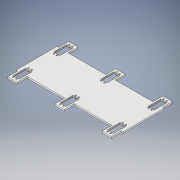
# Autodesk Inventor part: Body_Top
Saved by Autodesk Inventor 2017 (Build 210142000, 142)
## iProperties
Created: 2017-01-25
Part Number: Body_Top
Material: Generic
Document SubType Name: Modeling
Designer: Alexander Miller
Density: 1 g/cm^3
Appearance: Default
material_thickness: 5,000 mm
body_width: 130,000 mm
leg_distance: 120,000 mm
Author: Alexander Miller
Autodesk Inventor part; units mm, degrees
ref_plane "YZ Plane" through (0, 0, 0) normal (1, 0, 0) x (0, 1, 0)
ref_plane "XZ Plane" through (0, 0, 0) normal (0, 1, 0) x (-1, 0, 0)
ref_plane "XY Plane" through (0, 0, 0) normal (0, 0, 1) x (1, 0, 0)
sketch "Sketch1" plane through (0, 0, 0) normal (0, 1, 0) x (-1, 0, 0)
  line L0 (-170, 0) -> (-170, -65)
  line L1 (-170, -65) -> (-165, -65)
  line L2 (-165, -65) -> (-165, -96.75)
  line L3 (-165, -96.75) -> (-135, -96.75)
  line L4 (-135, -96.75) -> (-135, -65)
  line L5 (-135, -65) -> (-15, -65)
  line L6 (-15, -65) -> (-15, -96.75)
  line L7 (-15, -96.75) -> (15, -96.75)
  line L8 (15, -96.75) -> (15, -65)
  line L9 (15, -65) -> (135, -65)
  line L10 (135, -65) -> (135, -96.75)
  line L11 (135, -96.75) -> (165, -96.75)
  line L12 (165, -96.75) -> (165, -65)
  line L13 (165, -65) -> (170, -65)
  line L14 (170, -65) -> (170, 0)
  line L15 (238, 0) -> (-238, 0) projected
  line L16 (-170, 0) -> (-170, 65)
  line L17 (-170, 65) -> (-165, 65)
  line L18 (-165, 65) -> (-165, 96.75)
  line L19 (-165, 96.75) -> (-135, 96.75)
  line L20 (-135, 96.75) -> (-135, 65)
  line L21 (-135, 65) -> (-15, 65)
  line L22 (-15, 65) -> (-15, 96.75)
  line L23 (-15, 96.75) -> (15, 96.75)
  line L24 (15, 96.75) -> (15, 65)
  line L25 (15, 65) -> (135, 65)
  line L26 (135, 65) -> (135, 96.75)
  line L27 (135, 96.75) -> (165, 96.75)
  line L28 (165, 96.75) -> (165, 65)
  line L29 (165, 65) -> (170, 65)
  line L30 (170, 65) -> (170, 0)
  point P0 (0, 0)
  point P1 (0, -96.75)
  dimension "d0" = 30
  dimension "d1" = 65
  dimension "d2" = 31.75
  dimension "d3" = 5
  dimension "d4" = 120
  constraints: 60 end point, 18 point on line, 14 symmetric about line, 9 perpendicular, 5 equal length, 2 vertical, 1 horizontal alignment, 1 midpoint, 1 vertical alignment
  measures "d0" distance of L10.end L11.end
  measures "d1" distance of L13.end L14.end
  measures "d2" distance of L11.end L12.end
  measures "d3" distance of L12.end L13.end
  measures "d4" distance of L8.end L9.end
extrude "Extrusion1" add sketch "Sketch1" along normal blind 5
sketch "Sketch2" plane through (0, 5, 0) normal (0, 1, 0) x (1, 0, 0)
  line L0 (-140, 44.75) -> (-160, 44.75)
  line L1 (-160, 44.75) -> (-160, 85.25)
  line L2 (-160, 85.25) -> (-140, 85.25)
  line L3 (-140, 85.25) -> (-140, 44.75)
  line L4 (10, 44.75) -> (-10, 44.75)
  line L5 (-10, 44.75) -> (-10, 85.25)
  line L6 (-10, 85.25) -> (10, 85.25)
  line L7 (10, 85.25) -> (10, 44.75)
  line L8 (160, 44.75) -> (140, 44.75)
  line L9 (140, 44.75) -> (140, 85.25)
  line L10 (140, 85.25) -> (160, 85.25)
  line L11 (160, 85.25) -> (160, 44.75)
  line L12 (-238, 0) -> (238, 0) projected
  line L13 (-140, -44.75) -> (-160, -44.75)
  line L14 (-160, -44.75) -> (-160, -85.25)
  line L15 (-160, -85.25) -> (-140, -85.25)
  line L16 (-140, -85.25) -> (-140, -44.75)
  line L17 (10, -44.75) -> (-10, -44.75)
  line L18 (-10, -44.75) -> (-10, -85.25)
  line L19 (-10, -85.25) -> (10, -85.25)
  line L20 (10, -85.25) -> (10, -44.75)
  line L21 (160, -44.75) -> (140, -44.75)
  line L22 (140, -44.75) -> (140, -85.25)
  line L23 (140, -85.25) -> (160, -85.25)
  line L24 (160, -85.25) -> (160, -44.75)
  line L25 (-135, 96.75) -> (-165, 96.75) projected
  line L26 (-165, 96.75) -> (-165, 65) projected
  line L27 (-15, 96.75) -> (-15, 65) projected
  line L28 (135, 96.75) -> (135, 65) projected
  point P0 (0, 0)
  dimension "d7" = 11.5
  dimension "d8" = 5
  dimension "d9" = 20
  dimension "d10" = 40.5
  dimension "d11" = 5
  dimension "d12" = 5
  constraints: 48 end point, 12 symmetric about line, 6 parallel, 4 point on line, 3 horizontal, 3 perpendicular, 2 collinear, 2 horizontal alignment
  measures "d7" distance between parallel lines of L2 L25
  measures "d8" distance between parallel lines of L1 L26
  measures "d9" distance of L1.end L2.end
  measures "d10" distance of L2.end L0.start
  measures "d11" distance between parallel lines of L27 L5
  measures "d12" distance between parallel lines of L9 L28
extrude "Extrusion2" cut sketch "Sketch2" against normal through all
sketch "Sketch3" plane through (0, 5, 0) normal (0, 1, 0) x (1, 0, 0)
  circle A0 centre (-155, 40.75) radius 2.25
  circle A1 centre (-145, 40.75) radius 2.25
  circle A2 centre (-155, 89.25) radius 2.25
  circle A3 centre (-145, 89.25) radius 2.25
  circle A4 centre (-5, 40.75) radius 2.25
  circle A5 centre (-5, 89.25) radius 2.25
  line L0 (-135, 96.75) -> (-165, 96.75) projected
  line L1 (-160, 85.25) -> (-140, 85.25) projected
  line L2 (-140, 44.75) -> (-160, 44.75) projected
  line L3 (-160, 44.75) -> (-160, 85.25) projected
  line L4 (-140, 85.25) -> (-140, 44.75) projected
  line L5 (-10, 44.75) -> (-10, 85.25) projected
  line L6 (-238, 0) -> (238, 0) projected
  line L7 (0, 135.45) -> (0, -135.45) projected
  circle A6 centre (-155, -40.75) radius 2.25
  circle A7 centre (-145, -40.75) radius 2.25
  circle A8 centre (-155, -89.25) radius 2.25
  circle A9 centre (-145, -89.25) radius 2.25
  circle A10 centre (-5, -40.75) radius 2.25
  circle A11 centre (-5, -89.25) radius 2.25
  circle A12 centre (155, 40.75) radius 2.25
  circle A13 centre (145, 40.75) radius 2.25
  circle A14 centre (155, 89.25) radius 2.25
  circle A15 centre (145, 89.25) radius 2.25
  circle A16 centre (5, 40.75) radius 2.25
  circle A17 centre (5, 89.25) radius 2.25
  circle A18 centre (155, -40.75) radius 2.25
  circle A19 centre (145, -40.75) radius 2.25
  circle A20 centre (5, -40.75) radius 2.25
  circle A21 centre (5, -89.25) radius 2.25
  circle A22 centre (145, -89.25) radius 2.25
  circle A23 centre (155, -89.25) radius 2.25
  point P0 (0, 0)
  dimension "d17" = 4
  dimension "d18" = 4
  dimension "d19" = 4.5
  dimension "d25" = 2.75
  dimension "d26" = 2.75
  dimension "d27" = 2.75
  constraints: 24 centre point, 18 symmetric about line, 5 equal radius, 4 horizontal alignment, 3 vertical alignment, 18 other
  measures "d17" distance from line of L1 A2.centre
  measures "d18" distance from line of L2 A0.centre
  measures "d19" diameter of A2
  measures "d25" distance edge to line of A2 L3
  measures "d26" distance edge to line of A3 L4
  measures "d27" distance edge to line of A5 L5
extrude "Extrusion3" cut sketch "Sketch3" against normal through all contours A0 | A1 | A2 | A3 | A4 | A5 | A6 | A7 | A8 | A9 | A10 | A11 | A12 | A13 | A14 | A15 | A16 | A17 | A18 | A19 | A20 | A21 | A22 | A23
sketch "Sketch4" plane through (0, 0, 0) normal (0, -1, 0) x (1, 0, 0)
  line L0 (150.6, 91.75) -> (149.4, 91.75)
  line L1 (149.4, 91.75) -> (149.4, 85.25)
  line L2 (149.4, 85.25) -> (150.6, 85.25)
  line L3 (150.6, 85.25) -> (150.6, 91.75)
  line L4 (150.6, 44.75) -> (149.4, 44.75)
  line L5 (149.4, 44.75) -> (149.4, 38.25)
  line L6 (149.4, 38.25) -> (150.6, 38.25)
  line L7 (150.6, 38.25) -> (150.6, 44.75)
  line L8 (0.6, 91.75) -> (-0.6, 91.75)
  line L9 (-0.6, 91.75) -> (-0.6, 85.25)
  line L10 (-0.6, 85.25) -> (0.6, 85.25)
  line L11 (0.6, 85.25) -> (0.6, 91.75)
  line L12 (0.6, 44.75) -> (-0.6, 44.75)
  line L13 (-0.6, 44.75) -> (-0.6, 38.25)
  line L14 (-0.6, 38.25) -> (0.6, 38.25)
  line L15 (0.6, 38.25) -> (0.6, 44.75)
  line L16 (-149.4, 91.75) -> (-150.6, 91.75)
  line L17 (-150.6, 91.75) -> (-150.6, 85.25)
  line L18 (-150.6, 85.25) -> (-149.4, 85.25)
  line L19 (-149.4, 85.25) -> (-149.4, 91.75)
  line L20 (-149.4, 44.75) -> (-150.6, 44.75)
  line L21 (-150.6, 44.75) -> (-150.6, 38.25)
  line L22 (-150.6, 38.25) -> (-149.4, 38.25)
  line L23 (-149.4, 38.25) -> (-149.4, 44.75)
  line L24 (140, 85.25) -> (160, 85.25) projected
  line L25 (160, 44.75) -> (140, 44.75) projected
  line L26 (10, 44.75) -> (-10, 44.75) projected
  line L27 (-10, 85.25) -> (10, 85.25) projected
  line L28 (-160, 85.25) -> (-140, 85.25) projected
  line L29 (-140, 44.75) -> (-160, 44.75) projected
  line L30 (-238, 0) -> (238, 0) projected
  line L31 (150.6, -91.75) -> (149.4, -91.75)
  line L32 (149.4, -91.75) -> (149.4, -85.25)
  line L33 (149.4, -85.25) -> (150.6, -85.25)
  line L34 (150.6, -85.25) -> (150.6, -91.75)
  line L35 (150.6, -44.75) -> (149.4, -44.75)
  line L36 (149.4, -44.75) -> (149.4, -38.25)
  line L37 (149.4, -38.25) -> (150.6, -38.25)
  line L38 (150.6, -38.25) -> (150.6, -44.75)
  line L39 (0.6, -91.75) -> (-0.6, -91.75)
  line L40 (-0.6, -91.75) -> (-0.6, -85.25)
  line L41 (-0.6, -85.25) -> (0.6, -85.25)
  line L42 (0.6, -85.25) -> (0.6, -91.75)
  line L43 (0.6, -44.75) -> (-0.6, -44.75)
  line L44 (-0.6, -44.75) -> (-0.6, -38.25)
  line L45 (-0.6, -38.25) -> (0.6, -38.25)
  line L46 (0.6, -38.25) -> (0.6, -44.75)
  line L47 (-149.4, -91.75) -> (-150.6, -91.75)
  line L48 (-150.6, -91.75) -> (-150.6, -85.25)
  line L49 (-150.6, -85.25) -> (-149.4, -85.25)
  line L50 (-149.4, -85.25) -> (-149.4, -91.75)
  line L51 (-149.4, -44.75) -> (-150.6, -44.75)
  line L52 (-150.6, -44.75) -> (-150.6, -38.25)
  line L53 (-150.6, -38.25) -> (-149.4, -38.25)
  line L54 (-149.4, -38.25) -> (-149.4, -44.75)
  point P0 (0, 0)
  point P1 (150, 85.25)
  point P2 (150, 85.25)
  point P3 (150, 44.75)
  point P4 (150, 44.75)
  point P5 (0, 85.25)
  point P6 (0, 85.25)
  point P7 (0, 44.75)
  point P8 (0, 44.75)
  point P9 (-150, 85.25)
  point P10 (-150, 85.25)
  point P11 (-150, 44.75)
  point P12 (-150, 85.25)
  point P13 (150, -85.25)
  point P14 (150, -85.25)
  point P15 (150, -44.75)
  point P16 (150, -44.75)
  point P17 (0, -85.25)
  point P18 (0, -85.25)
  point P19 (0, -44.75)
  point P20 (0, -44.75)
  point P21 (-150, -85.25)
  point P22 (-150, -85.25)
  point P23 (-150, -44.75)
  point P24 (-150, -85.25)
  dimension "d30" = 6.5
  dimension "d31" = 1.2
  constraints: 96 end point, 36 symmetric about line, 12 midpoint, 12 parallel, 10 equal length, 6 collinear, 6 horizontal, 6 perpendicular, 5 coincident, 1 vertical alignment
  measures "d30" distance of L2.end L0.start
  measures "d31" distance of L0.start L0.end
extrude "Extrusion4" cut sketch "Sketch4" against normal blind 2
equation "\"d0\" = servo_depth + 2 * material_thickness"
equation "\"d1\" = 0.5 * body_width"
equation "\"d2\" = servo_mount_length + 0.5 * servo_width + material_thickness"
equation "\"d4\" = leg_distance"
equation "\"d5\" = material_thickness"
equation "\"d7\" = material_thickness + servo_mount_length"
equation "\"d8\" = material_thickness"
equation "\"d9\" = servo_depth"
equation "\"d10\" = servo_width"
equation "\"d11\" = d8"
equation "\"d12\" = d8"
equation "\"d13\" = material_thickness"
equation "\"d17\" = servo_mount_length - servo_mount_hole_front_distance"
equation "\"d18\" = d17"
equation "\"d19\" = servo_mount_hole_diameter"
equation "\"d25\" = servo_mount_hole_side_distance"
equation "\"d26\" = d25"
equation "\"d27\" = d25"
equation "\"d28\" = material_thickness"
equation "\"d30\" = servo_mount_length"
equation "\"d31\" = servo_mount_pin_thickness"
equation "\"d32\" = servo_mount_pin_height"
equation "\"material_thickness\" = 5"
equation "\"body_width\" = 130"
equation "\"leg_distance\" = 120"
equation "\"servo_depth\" = 20"
equation "\"servo_mount_length\" = 6.5"
equation "\"servo_width\" = 40.5"
equation "\"servo_mount_hole_front_distance\" = 2.5"
equation "\"servo_mount_hole_diameter\" = 4.5"
equation "\"servo_mount_hole_side_distance\" = 2.75"
equation "\"servo_mount_pin_thickness\" = 1.2"
equation "\"servo_mount_pin_height\" = 2"
body "Solid1"
